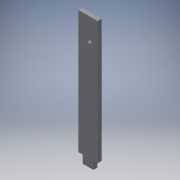
# Autodesk Inventor part: table_foot
Saved by Autodesk Inventor 2019.4 (Build 234330000, 330)
## iProperties
Created: 2019-12-14
Part Number: table_foot
Material: Generic
Document SubType Name: Modeling
Designer: fabfarm
Density: 1 g/cm^3
Appearance: Default
Author: fabfarm
Autodesk Inventor part; units mm, degrees
ref_plane "YZ Plane" through (0, 0, 0) normal (1, 0, 0) x (0, 1, 0)
ref_plane "XZ Plane" through (0, 0, 0) normal (0, 1, 0) x (-1, 0, 0)
ref_plane "XY Plane" through (0, 0, 0) normal (0, 0, 1) x (1, 0, 0)
sketch "Sketch1" plane through (0, 0, 0) normal (0, 0, 1) x (1, 0, 0)
  line L0 (0, 0) -> (0, 575)
  line L1 (0, 575) -> (90, 575)
  line L2 (90, 575) -> (90, 0)
  line L3 (90, 0) -> (0, 0)
  dimension "d0" = 575
  dimension "d1" = 90
  constraints: 8 end point, 3 perpendicular, 1 vertical
  measures "d0" distance of L1.end L2.end
  measures "d1" distance of L2.end L0.start
extrude "Extrusion1" add sketch "Sketch1" along normal blind 18.55
sketch "Sketch2" plane through (0, 0, 18.55) normal (0, 0, 1) x (1, 0, 0)
  circle A0 centre (50, 475) radius 10
  line L0 (0, 575) -> (0, 0) projected
  line L1 (0, 475) -> (90, 475) construction
  line L2 (90, 0) -> (90, 575) projected
  line L3 (90, 575) -> (0, 575) projected
  dimension "d4" = 50
  dimension "d5" = 100
  dimension "d6" = 20
  constraints: 3 point on line, 2 end point, 1 centre point, 1 horizontal
  measures "d4" distance from line of L0 A0.centre
  measures "d5" distance between parallel lines of L3 L1
  measures "d6" diameter of A0
extrude "Extrusion2" cut sketch "Sketch2" against normal blind 100
sketch "Sketch3" plane through (0, 0, 18.55) normal (0, 0, 1) x (1, 0, 0)
  line L0 (0, 0) -> (90, 0) projected
  line L1 (20, 0) -> (70, 0)
  line L2 (70, 0) -> (70, -37.1)
  line L3 (70, -37.1) -> (20, -37.1)
  line L4 (20, -37.1) -> (20, 0)
  line L5 (0, 575) -> (0, 0) projected
  line L6 (90, 0) -> (90, 575) projected
  dimension "d9" = 20
  dimension "d10" = 20
  dimension "d11" = 37.1
  constraints: 8 end point, 2 parallel, 1 horizontal, 1 perpendicular, 1 point on line
  measures "d9" distance between parallel lines of L5 L4
  measures "d10" distance between parallel lines of L2 L6
  measures "d11" distance of L1.end L2.end
extrude "Extrusion3" add sketch "Sketch3" against normal blind 18.55
sketch "Sketch4" plane through (0, 0, 18.55) normal (0, 0, 1) x (1, 0, 0)
  line L0 (35.7, 275) -> (54.3, 275)
  line L1 (54.3, 275) -> (54.3, 225)
  line L2 (54.3, 225) -> (35.7, 225)
  line L3 (35.7, 225) -> (35.7, 275)
  line L4 (90, 575) -> (0, 575) projected
  line L5 (35.7, 250) -> (0, 250) construction
  line L6 (0, 575) -> (0, 0) projected
  line L7 (54.3, 250) -> (90, 250) construction
  line L8 (90, 0) -> (90, 575) projected
  dimension "d14" = 300
  dimension "d15" = 50
  dimension "d16" = 18.6
  constraints: 12 end point, 3 horizontal, 2 midpoint, 2 parallel, 2 point on line, 1 collinear, 1 perpendicular
  measures "d14" distance between parallel lines of L4 L0
  measures "d15" distance of L2.end L0.start
  measures "d16" distance of L1.end L2.end
extrude "Extrusion4" cut sketch "Sketch4" against normal blind 200
body "Solid1"
